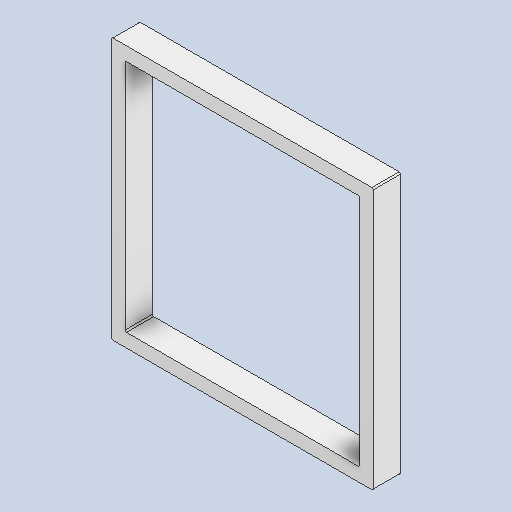
# Autodesk Inventor part: infTrim
Saved by Autodesk Inventor 2023 (Build 270158000, 158)
## iProperties
Created: 2024-05-07
Part Number: infTrim
Material: ABS Plastic
Document SubType Name: Modeling
Designer: jonwo
Density: 1.06 g/cm^3
Appearance: Smooth - White
Author: jonwo
Autodesk Inventor part; units mm, degrees
ref_plane "YZ Plane" through (0, 0, 0) normal (1, 0, 0) x (0, 1, 0)
ref_plane "XZ Plane" through (0, 0, 0) normal (0, 1, 0) x (-1, 0, 0)
ref_plane "XY Plane" through (0, 0, 0) normal (0, 0, 1) x (1, 0, 0)
sketch "Sketch1" plane through (0, 0, 0) normal (0, 0, 1) x (1, 0, 0)
  line L0 (-36.576, 56.9271) -> (-36.576, 8.1591) projected
  line L1 (-36.576, 8.1591) -> (12.192, 8.1591) projected
  line L2 (12.192, 8.1591) -> (12.192, 56.9271) projected
  line L3 (12.192, 56.9271) -> (-36.576, 56.9271) projected
  line L4 (9.652, 10.6991) -> (-34.036, 10.6991)
  line L5 (-34.036, 10.6991) -> (-34.036, 54.3871)
  line L6 (-34.036, 54.3871) -> (9.652, 54.3871)
  line L7 (9.652, 54.3871) -> (9.652, 10.6991)
  point P0 (0, 0)
  dimension "d0" = 2.54
  constraints: 8 end point, 3 other
  measures "d0" distance between parallel lines of L1 L4
extrude "Extrusion1" add sketch "Sketch1" along normal blind 5.08
fillet "Fillet1" radius 0.254 8 edges at (12.192, 8.1591, 2.54) (-36.576, 8.1591, 2.54) (-36.576, 56.9271, 2.54) (12.192, 56.9271, 2.54) (-34.036, 10.6991, 2.54) (9.652, 10.6991, 2.54) (-34.036, 54.3871, 2.54) (9.652, 54.3871, 2.54)
body "Solid1"
